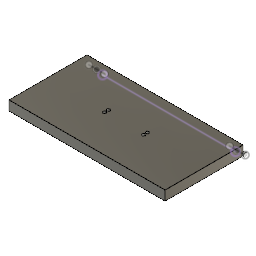
Semana4_Desafio6 (montagem) v2 (Autodesk Fusion 360 archive; units mm, degrees)
design "Semana4_Desafio6 (tampa)"
Autodesk Fusion 360 part; units mm, degrees
sketch "Sketch1" plane through (0, 0, 0) normal (0, 0, 1) x (1, 0, 0)
  line L0 (200, -100) -> (-200, -100)
  line L1 (-200, -100) -> (-200, 100)
  line L2 (-200, 100) -> (200, 100)
  line L3 (200, 100) -> (200, -100)
  line L4 (200, -100) -> (-200, 100) construction
  line L5 (-200, -100) -> (200, 100) construction
  line L6 (195, -95) -> (-195, -95)
  line L7 (-195, -95) -> (-195, 95)
  line L8 (-195, 95) -> (195, 95)
  line L9 (195, 95) -> (195, -95)
  line L10 (195, -95) -> (-195, 95) construction
  line L11 (-195, -95) -> (195, 95) construction
  dimension "d1" = 400
  dimension "d2" = 200
  dimension "d3" = 390
  dimension "d4" = 190
  constraint horizontal L0
  constraint perpendicular L0 L1
  constraint parallel L0 L2
  constraint parallel L1 L3
  constraint coincident L4 origin
  constraint coincident L5 origin
  constraint horizontal L6
  constraint perpendicular L6 L7
  constraint parallel L6 L8
  constraint parallel L7 L9
  constraint coincident L10 origin
  constraint coincident L11 origin
  measures "d1" distance of L1.end L2.end
  measures "d2" distance of L0.end L1.end
  measures "d3" distance of L7.end L8.end
  measures "d4" distance of L6.end L7.end
extrude "Extrude1" add sketch "Sketch1" along normal blind 25
sketch "Sketch2" plane through (0, 0, 25) normal (0, 0, 1) x (-1, 0, 0)
  line L0 (195, -95) -> (-195, -95)
  line L1 (-195, -95) -> (-195, 95)
  line L2 (-195, 95) -> (195, 95)
  line L3 (195, 95) -> (195, -95)
  line L4 (-200, -100) -> (200, -100)
  line L5 (200, -100) -> (200, 100)
  line L6 (200, 100) -> (-200, 100)
  line L7 (-200, 100) -> (-200, -100)
  line L8 (-200, 100) -> (200, 100)
  line L9 (200, 100) -> (200, -100)
  line L10 (200, -100) -> (-200, -100)
  line L11 (-200, -100) -> (-200, 100)
  line L12 (-200, 100) -> (200, -100) construction
  line L13 (200, 100) -> (-200, -100) construction
  constraint horizontal L8
  constraint perpendicular L8 L9
  constraint parallel L8 L10
  constraint parallel L9 L11
  constraint coincident L6.end L7.start
  constraint coincident L12 origin
  constraint coincident L13 origin
extrude "Extrude2" add sketch "Sketch2" against normal blind 10 contours L0 L1 L2 L3
sketch "Sketch3" plane through (0, 0, 0) normal (0, 0, -1) x (1, 0, 0)
  line L0 (195, -95) -> (-195, -95)
  line L1 (-195, -95) -> (-195, 95)
  line L2 (-195, 95) -> (195, 95)
  line L3 (195, 95) -> (195, -95)
  line L4 (-200, -100) -> (200, -100)
  line L5 (200, -100) -> (200, 100)
  line L6 (200, 100) -> (-200, 100)
  line L7 (-200, 100) -> (-200, -100)
  line L8 (200, -100) -> (200, -97.5)
  line L9 (200, -97.5) -> (180, -97.5)
  line L10 (180, -97.5) -> (180, -100)
  line L11 (200, -100) -> (180, -100)
  line L12 (-180, -100) -> (-180, -97.5)
  line L13 (-180, -97.5) -> (-160, -97.5)
  line L14 (-160, -97.5) -> (-160, -100)
  line L15 (-160, -100) -> (-180, -100)
  dimension "d9" = 2.5
  dimension "d11" = 20
  dimension "d12" = 2.5
  dimension "d13" = 20
  dimension "d14" = 20
  constraint coincident L4 L5.start
  constraint perpendicular L0 L8
  constraint perpendicular L8 L9
  constraint coincident L4 L10.end
  constraint perpendicular L4 L10
  constraint collinear L5 L8
  constraint coincident L4 L12.start
  constraint perpendicular L4 L12
  constraint perpendicular L12 L13
  constraint coincident L4 L14.end
  constraint perpendicular L4 L14
  measures "d9" distance of L4.end L8.end
  measures "d11" distance of L8 L10
  measures "d12" distance of L12.start L12.end
  measures "d13" distance of L12.end L13.end
  measures "d14" distance of L7 L12
extrude "Extrude3" cut sketch "Sketch3" against normal blind 7.5 contours L4 L12 L13 L14 L15 | L4 L5 L8 L9 L10 L11
sketch "Sketch4" plane through (0, 0, 0) normal (0, 0, 1) x (1, 0, 0)
  line L0 (200, 105) -> (160, 105)
  line L1 (-160.0025, 105) -> (-199.9975, 105)
  line L2 (-160, 100) -> (180, 100)
  point P0 (-180, 105)
  point P1 (180, 105)
  dimension "d17" = 5
  constraint horizontal L0
  constraint horizontal L1
  constraint midpoint L1 P0
  constraint midpoint L0 P1
  constraint horizontal P0 P1
  measures "d17" distance of L0 L2
pipe "Pipe1" add diameter 10 path "Sketch4" along L0
pipe "Pipe2" add diameter 10 path "Sketch4" along L1
fillet "Fillet1" radius 0.5 1 edges at (200, 109.6616, -1.8081)
fillet "Fillet2" radius 0.5 1 edges at (-160.0025, 109.6616, -1.8081)
sketch "Sketch7" plane through (0, 0, 15) normal (0, 0, -1) x (1, 0, 0)
  line L0 (195, 95) -> (-195, 95)
  line L1 (-195, 95) -> (-195, -95)
  line L2 (-195, -95) -> (195, -95)
  line L3 (195, -95) -> (195, 95)
  line L4 (-55, 10) -> (-55, -10) construction
  line L5 (-55, -10) -> (-45, -10) construction
  line L6 (-45, -10) -> (-45, 10) construction
  line L7 (-45, 10) -> (-55, 10) construction
  line L8 (55, 0) -> (55, 10) construction
  line L9 (55, 10) -> (45, 10) construction
  line L10 (45, 10) -> (45, -10) construction
  line L11 (45, -10) -> (55, -10) construction
  line L12 (55, -10) -> (55, 0) construction
  circle A0 centre (50, 5) radius 4
  circle A1 centre (50, -5) radius 4
  circle A2 centre (-50, 5) radius 4
  circle A3 centre (-50, -5) radius 4
  dimension "d64" = 8
  dimension "d65" = 8
  dimension "d66" = 8
  dimension "d67" = 8
  constraint vertical L4
  constraint perpendicular L4 L5
  constraint perpendicular L5 L6
  constraint perpendicular L6 L7
  constraint vertical L8
  constraint perpendicular L8 L9
  constraint perpendicular L9 L10
  constraint perpendicular L10 L11
  constraint perpendicular L11 L12
  measures "d64" diameter of A0
  measures "d65" diameter of A1
  measures "d66" diameter of A2
  measures "d67" diameter of A3
extrude "Extrude5" cut sketch "Sketch7" against normal blind 10 contours A0 | A1 | A2 | A3

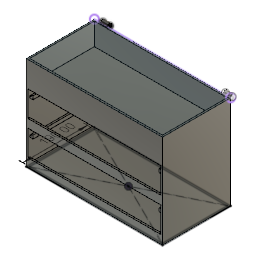
design "Semana4_Desafio6 (Estrutura)"
Autodesk Fusion 360 part; units mm, degrees
sketch "Sketch1" plane through (0, 0, 0) normal (0, 0, 1) x (1, 0, 0)
  line L0 (200, -100) -> (-200, -100)
  line L1 (-200, -100) -> (-200, 100)
  line L2 (-200, 100) -> (200, 100)
  line L3 (200, 100) -> (200, -100)
  line L4 (200, -100) -> (-200, 100) construction
  line L5 (-200, -100) -> (200, 100) construction
  line L6 (195, -95) -> (-195, -95)
  line L7 (-195, -95) -> (-195, 95)
  line L8 (-195, 95) -> (195, 95)
  line L9 (195, 95) -> (195, -95)
  line L10 (195, -95) -> (-195, 95) construction
  line L11 (-195, -95) -> (195, 95) construction
  dimension "d1" = 200
  dimension "d2" = 400
  dimension "d3" = 390
  dimension "d4" = 190
  constraint horizontal L0
  constraint perpendicular L0 L1
  constraint parallel L0 L2
  constraint parallel L1 L3
  constraint coincident L4 origin
  constraint coincident L5 origin
  constraint horizontal L6
  constraint perpendicular L6 L7
  constraint parallel L6 L8
  constraint parallel L7 L9
  constraint coincident L10 origin
  constraint coincident L11 origin
  measures "d1" distance of L0.end L1.end
  measures "d2" distance of L1.end L2.end
  measures "d3" distance of L7.end L8.end
  measures "d4" distance of L6.end L7.end
extrude "Extrude1" add sketch "Sketch1" along normal blind 275
sketch "Sketch3" plane through (0, -100, 0) normal (0, -1, 0) x (1, 0, 0)
  line L0 (-200, 0) -> (200, 0)
  line L1 (200, 0) -> (200, 275)
  line L2 (200, 275) -> (-200, 275)
  line L3 (-200, 275) -> (-200, 0)
  line L4 (-195, 200) -> (195, 200)
  line L5 (195, 200) -> (195, 125)
  line L6 (195, 125) -> (-195, 125)
  line L7 (-195, 125) -> (-195, 200)
  line L8 (-195, 100) -> (195, 100)
  line L9 (195, 100) -> (195, 25)
  line L10 (195, 25) -> (-195, 25)
  line L11 (-195, 25) -> (-195, 100)
  line L12 (200, 0) -> (-200, 0)
  dimension "d11" = 5
  dimension "d12" = 5
  dimension "d13" = 25
  dimension "d14" = 25
  constraint horizontal L4
  constraint vertical L5
  constraint horizontal L6
  constraint vertical L7
  constraint horizontal L8
  constraint vertical L9
  constraint horizontal L10
  constraint vertical L11
  constraint collinear L7 L11
  constraint collinear L5 L9
  measures "d11" distance of L3 L7
  measures "d12" distance of L1 L5
  measures "d13" distance of L10 L12
  measures "d14" distance of L6 L8
extrude "Extrude2" cut sketch "Sketch3" against normal blind 10 contours L4 L5 L6 L7 | L8 L9 L10 L11
extrude "Extrude3" add sketch "Sketch1" along normal blind 10 contours L6 L7 L8 L9
ref_plane "WorkPlane1" through (0, 0, 200) normal (0, 0, 1) x (1, 0, 0)
sketch "Sketch4" plane through (0, 0, 200) normal (0, 0, 1) x (1, 0, 0)
  line L0 (200, -100) -> (-200, -100)
  line L1 (-200, -100) -> (-200, 100)
  line L2 (-200, 100) -> (200, 100)
  line L3 (200, 100) -> (200, -100)
  line L4 (200, -100) -> (-200, 100) construction
  line L5 (-200, -100) -> (200, 100) construction
  constraint horizontal L0
  constraint perpendicular L0 L1
  constraint parallel L0 L2
  constraint parallel L1 L3
  constraint coincident L4 origin
  constraint coincident L5 origin
extrude "Extrude4" add sketch "Sketch4" along normal blind 10
ref_plane "WorkPlane2" through (0, 0, 75) normal (0, 0, 1) x (1, 0, 0)
sketch "Sketch5" plane through (0, 0, 75) normal (0, 0, 1) x (1, 0, 0)
  line L0 (195, -95) -> (185, -95)
  line L1 (185, -95) -> (185, 95)
  line L2 (185, 95) -> (195, 95)
  line L3 (195, 95) -> (195, -95)
  line L4 (-195, -95) -> (-185, -95)
  line L5 (-185, -95) -> (-185, 95)
  line L6 (-185, 95) -> (-195, 95)
  line L7 (-195, 95) -> (-195, -95)
  line L8 (-190, -95) -> (-190, 95)
  line L9 (190, -95) -> (190, 95)
  line L10 (195, -95) -> (-195, -95)
  line L11 (-195, -95) -> (-195, 95)
  line L12 (-195, 95) -> (195, 95)
  line L13 (195, 95) -> (185, 95)
  line L14 (185, -95) -> (195, -95)
  dimension "d19" = 10
  dimension "d20" = 10
  dimension "d21" = 5
  dimension "d22" = 5
  constraint horizontal L0
  constraint vertical L1
  constraint horizontal L2
  constraint vertical L3
  constraint horizontal L4
  constraint vertical L5
  constraint horizontal L6
  constraint vertical L7
  constraint vertical L8
  constraint vertical L9
  constraint collinear L4 L10
  constraint coincident L8.start L10
  constraint collinear L2 L12
  constraint coincident L9.end L12
  constraint coincident L0.end L10
  constraint coincident L9.start L10
  constraint coincident L2.end L3.start
  measures "d19" distance of L0.start L0.end
  measures "d20" distance of L4.start L4.end
  measures "d21" distance of L8 L11
  measures "d22" distance of L1 L9
extrude "Extrude5" add sketch "Sketch5" along normal blind 5 contours L4 L6 L7 L8 L10 L11 L12
extrude "Extrude6" add sketch "Sketch5" along normal blind 5 contours L0 L2 L3 L9 L10 L12 L13 L14
extrude "Extrude7" add sketch "Sketch5" along normal blind 10 contours L0 L1 L2 L9 L10 L12 L13 L14 | L4 L5 L6 L8 L10 L12
ref_plane "WorkPlane3" through (0, 0, 175) normal (0, 0, 1) x (1, 0, 0)
sketch "Sketch6" plane through (0, 0, 175) normal (0, 0, 1) x (1, 0, 0)
  line L0 (-195, 95) -> (-185, 95)
  line L1 (-185, 95) -> (-185, -95)
  line L2 (-185, -95) -> (-195, -95)
  line L3 (-195, -95) -> (-195, 95)
  line L4 (-190, 95) -> (-190, -95)
  line L5 (-195, 95) -> (195, 95)
  line L6 (195, -95) -> (-195, -95)
  line L7 (195, -95) -> (185, -95)
  line L8 (185, -95) -> (185, 95)
  line L9 (185, 95) -> (195, 95)
  line L10 (195, 95) -> (195, -95)
  line L11 (190, 95) -> (190, -95)
  dimension "d30" = 5
  dimension "d31" = 5
  constraint horizontal L0
  constraint vertical L1
  constraint horizontal L2
  constraint vertical L3
  constraint vertical L4
  constraint collinear L0 L5
  constraint collinear L2 L6
  constraint coincident L4.start L5
  constraint coincident L4.end L6
  constraint midpoint L0 L4.start
  constraint horizontal L7
  constraint vertical L8
  constraint horizontal L9
  constraint vertical L10
  constraint coincident L5 L8.end
  constraint coincident L6.start L7.start
  constraint midpoint L9 L11.start
  constraint midpoint L7 L11.end
  constraint coincident L3 L0.start
  measures "d30" distance of L10 L11
  measures "d31" distance of L3 L4
extrude "Extrude8" add sketch "Sketch6" along normal blind 5 contours L0 L2 L3 L4 L5 L6 | L5 L6 L7 L9 L10 L11
extrude "Extrude9" add sketch "Sketch6" along normal blind 10 contours L0 L1 L2 L4 L5 L6 | L5 L6 L7 L8 L9 L11
sketch "Sketch7" plane through (0, 0, 275) normal (0, 0, 1) x (-1, 0, 0)
  line L0 (195, -95) -> (-195, -95)
  line L1 (-195, -95) -> (-195, 95)
  line L2 (-195, 95) -> (195, 95)
  line L3 (195, 95) -> (195, -95)
  line L4 (-200, -100) -> (200, -100)
  line L5 (200, -100) -> (200, 100)
  line L6 (200, 100) -> (-200, 100)
  line L7 (-200, 100) -> (-200, -100)
  line L8 (-179.6402, -105) -> (-199.6402, -105)
  line L9 (200, -100) -> (-200, -100)
  line L10 (180, -105) -> (160, -105)
  dimension "d36" = 5
  dimension "d37" = 5
  dimension "d50" = 20
  dimension "d51" = 20
  constraint parallel L4 L8
  constraint horizontal L10
  measures "d36" distance of L8 L9
  measures "d37" distance of L9 L10
  measures "d50" horizontal distance of L4.end L10.start
  measures "d51" distance of L10.start L10.end
pipe "Pipe2" add diameter 15 wall 2.5 path "Sketch7" along L10
pipe "Pipe3" add diameter 15 wall 2.5 path "Sketch7" along L8

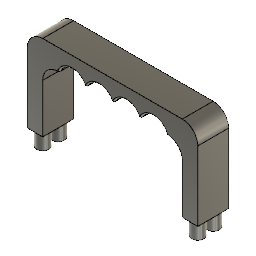
design "Semana4_Desafio6 (alça)"
Autodesk Fusion 360 part; units mm, degrees
sketch "Sketch1" plane through (0, 0, 0) normal (0, 1, 0) x (1, 0, 0)
  line L0 (-26.25, -38.343739) -> (-55, -38.343739) construction
  arc A0 (18.397436, -42.203757) -> (34.374038, -41.593739) centre (26.25, -38.343739) ccw
  arc A1 (45, -55) -> (55, -45) centre (45, -45) ccw
  line L1 (34.374038, -41.593739) -> (35, -41.593739)
  arc A2 (0.897436, -42.203757) -> (-0.897436, -42.203757) centre (0, -42.644901) ccw
  arc A3 (18.397436, -42.203757) -> (16.602564, -42.203757) centre (17.5, -42.644901) ccw
  arc A4 (-34.374038, -41.593739) -> (-18.397436, -42.203757) centre (-26.25, -38.343739) ccw
  arc A5 (-55, -45) -> (-45, -55) centre (-45, -45) ccw
  line L2 (-35, -29.593739) -> (35, -29.593739) construction
  line L3 (45, -45) -> (18.125962, -41.593739) construction
  arc A6 (0.897436, -42.203757) -> (16.602564, -42.203757) centre (8.75, -38.343739) ccw
  line L4 (45, -55) -> (-45, -55)
  line L5 (-34.374038, -41.593739) -> (-45, -45) construction
  line L6 (26.25, -38.343739) -> (55, -38.343739) construction
  arc A7 (-45, -31.593739) -> (-35, -41.593739) centre (-35, -31.593739) ccw
  line L7 (0, 0) -> (0, -57.946001) construction
  arc A8 (-16.602564, -42.203757) -> (-18.397436, -42.203757) centre (-17.5, -42.644901) ccw
  arc A9 (-16.602564, -42.203757) -> (-0.897436, -42.203757) centre (-8.75, -38.343739) ccw
  arc A10 (35, -41.593739) -> (45, -31.593739) centre (35, -31.593739) ccw
  line L8 (-35, -41.593739) -> (-34.374038, -41.593739)
  line L9 (-55, -45) -> (-55, 0)
  line L10 (-55, 0) -> (-45, 0)
  line L11 (-45, 0) -> (-45, -31.593739)
  line L12 (55, -45) -> (55, 0)
  line L13 (55, 0) -> (45, 0)
  line L14 (45, 0) -> (45, -31.593739)
  line L15 (55, 0) -> (-55, 0) construction
  dimension "d1" = 10
  dimension "d2" = 10
  dimension "d3" = 10
  dimension "d4" = 17.5
  dimension "d5" = 17.5
  dimension "d6" = 17.5
  dimension "d7" = 17.5
  dimension "d8" = 17.5
  dimension "d9" = 17.5
  dimension "d10" = 17.5
  dimension "d11" = 12
  dimension "d12" = 1
  dimension "d13" = 1
  dimension "d14" = 1
  constraint tangent A5 L4
  constraint tangent A1 L4
  constraint tangent A7 L8
  constraint tangent A10 L8
  constraint equal A7 A10
  constraint coincident A1.centre L3.start
  constraint coincident A5.centre L5.end
  constraint parallel L2 L8
  constraint tangent A4 L2
  constraint tangent A0 L2
  constraint equal L0 L6
  constraint collinear L1 L8
  constraint tangent A4 A8
  constraint tangent A8 A9
  constraint tangent A2 A9
  constraint tangent A2 A6
  constraint tangent A3 A6
  constraint tangent A0 A3
  constraint vertical L7
  constraint tangent A5 L9
  constraint vertical L9
  constraint perpendicular L9 L10
  constraint tangent A7 L11
  constraint tangent A1 L12
  constraint perpendicular L6 L12
  constraint perpendicular L12 L13
  constraint tangent A10 L14
  constraint coincident L7.start origin
  constraint perpendicular L7 L15
  constraint collinear L10 L13
  constraint collinear L10 L15
  measures "d1" radius of A5
  measures "d2" radius of A1
  measures "d3" radius of A7
  measures "d4" diameter of A4
  measures "d5" diameter of A9
  measures "d6" diameter of A6
  measures "d7" diameter of A0
  measures "d11" distance of L2 L8
  measures "d12" radius of A8
  measures "d13" radius of A2
  measures "d14" radius of A3
extrude "Extrude1" add sketch "Sketch1" along normal mid plane 20 contours A0 A1 L1 A2 A3 A4 A5 A6 L4 A7 A8 A9 A10 L8 L9 L10 L11 L12 L13 L14 picked at (-51.666667, -25.531246)
fillet "Fillet1" radius 1 14 edges at (-26.583849, -10, 47.087368) (-17.5, -10, 41.644901) (-8.75, -10, 47.093739) (0, -10, 41.644901) (8.75, -10, 47.093739) (17.5, -10, 41.644901) (26.583849, -10, 47.087368) (26.583849, 10, 47.087368) (17.5, 10, 41.644901) (8.75, 10, 47.093739) (0, 10, 41.644901) (-8.75, 10, 47.093739) (-17.5, 10, 41.644901) (-26.583849, 10, 47.087368)
sketch "Sketch2" plane through (0, 0, 0) normal (0, 0, 1) x (1, 0, 0)
  circle A0 centre (-50, -5) radius 4
  circle A1 centre (-50, 5) radius 4
  circle A2 centre (50, -5) radius 4
  circle A3 centre (50, 5) radius 4
  dimension "d18" = 8
  dimension "d19" = 8
  dimension "d20" = 8
  dimension "d21" = 8
  measures "d18" diameter of A0
  measures "d19" diameter of A1
  measures "d20" diameter of A2
  measures "d21" diameter of A3
extrude "Extrude2" add sketch "Sketch2" against normal blind 10 contours A0 | A1 | A2 | A3 picked at (-51.229753, -5.198723) picked at (-51.229753, 4.801277) picked at (48.770247, -5.198723) picked at (48.770247, 4.801277)

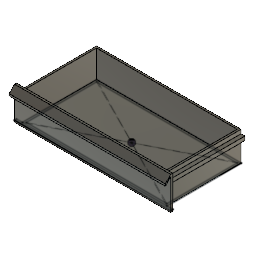
design "Semana4_Desafio6 (gaveta)"
Autodesk Fusion 360 part; units mm, degrees
sketch "Sketch1" plane through (0, 0, 0) normal (0, 0, 1) x (1, 0, 0)
  line L0 (185, -95) -> (-185, -95)
  line L1 (-185, -95) -> (-185, 95)
  line L2 (-185, 95) -> (185, 95)
  line L3 (185, 95) -> (185, -95)
  line L4 (185, -95) -> (-185, 95) construction
  line L5 (-185, -95) -> (185, 95) construction
  line L6 (180, -90) -> (-180, -90)
  line L7 (-180, -90) -> (-180, 90)
  line L8 (-180, 90) -> (180, 90)
  line L9 (180, 90) -> (180, -90)
  line L10 (180, -90) -> (-180, 90) construction
  line L11 (-180, -90) -> (180, 90) construction
  line L12 (-185, -95) -> (-200, -95)
  line L13 (-200, -95) -> (-200, -100)
  line L14 (-200, -100) -> (200, -100)
  line L15 (185, -95) -> (200, -95)
  line L16 (200, -95) -> (200, -100)
  dimension "d1" = 370
  dimension "d2" = 190
  dimension "d3" = 360
  dimension "d4" = 180
  dimension "d5" = 400
  dimension "d6" = 15
  dimension "d7" = 5
  constraint horizontal L0
  constraint perpendicular L0 L1
  constraint parallel L0 L2
  constraint parallel L1 L3
  constraint coincident L4 origin
  constraint coincident L5 origin
  constraint horizontal L6
  constraint perpendicular L6 L7
  constraint parallel L6 L8
  constraint parallel L7 L9
  constraint coincident L10 origin
  constraint coincident L11 origin
  constraint perpendicular L1 L12
  constraint perpendicular L12 L13
  constraint perpendicular L13 L14
  constraint perpendicular L3 L15
  constraint perpendicular L14 L16
  measures "d1" distance of L1.end L2.end
  measures "d2" distance of L0.end L1.end
  measures "d3" distance of L7.end L8.end
  measures "d4" distance of L6.end L7.end
  measures "d5" distance of L13.end L14.end
  measures "d6" distance of L0.start L15.end
  measures "d7" distance of L14.end L15.end
extrude "Extrude1" add sketch "Sketch1" along normal blind 75 contours L0 L1 L2 L3
extrude "Extrude2" add sketch "Sketch1" along normal blind 5 contours L6 L7 L8 L9
extrude "Extrude3" add sketch "Sketch1" along normal blind 80 and the other way blind 5 contours L0 L12 L13 L14 L15 L16
sketch "Sketch9" plane through (185, 0, 0) normal (1, 0, 0) x (0, 1, 0)
  line L0 (-95, 0) -> (95, 0)
  line L1 (95, 0) -> (95, 75)
  line L2 (95, 75) -> (-95, 75)
  line L3 (-95, 75) -> (-95, 0)
  line L4 (0, 0) -> (0, 60) construction
  line L5 (0, 60) -> (95, 60) construction
  line L6 (0, 60) -> (-95, 60) construction
  line L7 (-95, 60) -> (95, 60)
  line L8 (95, 60) -> (95, 65)
  line L9 (95, 65) -> (-95, 65)
  line L10 (-95, 65) -> (-95, 60)
  dimension "d48" = 5
  dimension "d49" = 60
  constraint coincident L4.start origin
  constraint perpendicular L0 L4
  constraint coincident L1 L5.end
  constraint perpendicular L1 L5
  constraint coincident L3 L6.end
  constraint perpendicular L3 L6
  constraint horizontal L7
  constraint vertical L8
  constraint horizontal L9
  constraint vertical L10
  measures "d48" distance of L6.end L9.end
  measures "d49" distance of L4.start L4.end
extrude "Extrude10" add sketch "Sketch9" along normal blind 10 contours L1 L3 L7 L8 L9 L10
sketch "Sketch10" plane through (0, 0, 60) normal (0, 0, -1) x (1, 0, 0)
  line L0 (185, 95) -> (185, -95)
  line L1 (185, -95) -> (195, -95)
  line L2 (195, -95) -> (195, 95)
  line L3 (195, 95) -> (185, 95)
  line L4 (195, -95) -> (190, -95)
  line L5 (190, -95) -> (190, 95)
  line L6 (190, 95) -> (195, 95)
  line L7 (195, 95) -> (195, -95)
  constraint horizontal L4
  constraint vertical L5
  constraint horizontal L6
  constraint vertical L7
  constraint midpoint L3 L5.end
  constraint coincident L1.end L2.start
extrude "Extrude11" add sketch "Sketch10" along normal blind 5 contours L1 L2 L3 L4 L5 L6 L7
sketch "Sketch11" plane through (-185, 0, 0) normal (-1, 0, 0) x (0, -1, 0)
  line L0 (-95, 0) -> (95, 0)
  line L1 (95, 0) -> (95, 75)
  line L2 (95, 75) -> (-95, 75)
  line L3 (-95, 75) -> (-95, 0)
  line L4 (0, 0) -> (0, 60) construction
  line L5 (95, 60) -> (-95, 60)
  line L6 (-95, 60) -> (-95, 65)
  line L7 (-95, 65) -> (95, 65)
  line L8 (95, 65) -> (95, 60)
  dimension "d54" = 5
  dimension "d55" = 190
  dimension "d56" = 60
  constraint coincident L4.start origin
  constraint perpendicular L0 L4
  constraint horizontal L5
  constraint vertical L6
  constraint horizontal L7
  constraint vertical L8
  constraint coincident L3 L6.end
  constraint coincident L4.end L5
  measures "d54" distance of L5.start L7.end
  measures "d55" distance of L6.end L7.end
  measures "d56" distance of L4.start L4.end
extrude "Extrude12" add sketch "Sketch11" along normal blind 10 contours L1 L3 L5 L6 L7 L8
sketch "Sketch13" plane through (0, 0, 60) normal (0, 0, -1) x (1, 0, 0)
  line L0 (-185, -95) -> (-185, 95)
  line L1 (-185, 95) -> (-195, 95)
  line L2 (-195, 95) -> (-195, -95)
  line L3 (-195, -95) -> (-185, -95)
  line L4 (-190, -95) -> (-195, -95)
  line L5 (-195, -95) -> (-195, 95)
  line L6 (-195, 95) -> (-190, 95)
  line L7 (-190, 95) -> (-190, -95)
  constraint horizontal L4
  constraint vertical L5
  constraint horizontal L6
  constraint vertical L7
  constraint coincident L1.end L2.start
  constraint midpoint L3 L4.start
extrude "Extrude13" add sketch "Sketch13" along normal blind 5 contours L1 L2 L3 L4 L5 L6 L7
sketch "Sketch14" plane through (0, 0, 0) normal (1, 0, 0) x (0, 1, 0)
  line L0 (-100, 80, -200) -> (-100, 80, 200)
  line L1 (-100, 80) -> (-114.1421, 65.8579)
  line L2 (-100, 80) -> (-120, 80) construction
  line L3 (-114.1421, 65.8579) -> (-114.1421, 60.8579)
  line L4 (-100, 80) -> (-100, 75)
  line L5 (-100, 75) -> (-114.1421, 60.8579)
  dimension "d61" = 45
  dimension "d62" = 20
  dimension "d63" = 5
  constraint horizontal L2
  constraint vertical L3
  constraint perpendicular L2 L4
  constraint parallel L1 L5
  measures "d61" angle of L1 L2
  measures "d62" distance of L1.start L1.end
  measures "d63" distance of L1.end L3.end
extrude "Extrude14" add sketch "Sketch14" along normal mid plane 400
